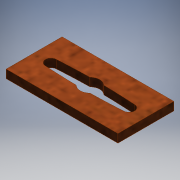
# Autodesk Inventor part: acople madera
Saved by Autodesk Inventor 2016 (Build 200138000, 138)
## iProperties
Created: 2016-08-02
Part Number: acople madera
Material: Madera (nogal)
Document SubType Name: Modeling
Designer: DanielFelipe
Density: 0.55 g/cm^3
Appearance: Nogal - Natural pulido
Mass: 1.07378 g
Surface Area: 18.7068 cm^2
Volume: 1.95232 cm^3
Author: DanielFelipe
Autodesk Inventor part; units mm, degrees
ref_plane "YZ Plane" through (0, 0, 0) normal (1, 0, 0) x (0, 1, 0)
ref_plane "XZ Plane" through (0, 0, 0) normal (0, 1, 0) x (-1, 0, 0)
ref_plane "XY Plane" through (0, 0, 0) normal (0, 0, 1) x (1, 0, 0)
sketch "Boceto1" plane through (0, 0, 0) normal (0, 0, 1) x (1, 0, 0)
  arc A0 (-2.4791, 2.4706) -> (-14, 2) centre (1.6231, -239.1959) ccw
  arc A1 (-14, 2) -> (-14, -2) centre (-14, 0) ccw
  arc A2 (-14, -2) -> (-2.4791, -2.4706) centre (1.6231, 239.1959) ccw
  arc A3 (2.4791, -2.4706) -> (14, -2) centre (-1.6231, 239.1959) ccw
  arc A4 (14, -2) -> (14, 2) centre (14, 0) ccw
  arc A5 (14, 2) -> (2.4791, 2.4706) centre (-1.6231, -239.1959) ccw
  line L0 (-20, -10) -> (20, -10)
  line L1 (20, -10) -> (20, 10)
  line L2 (20, 10) -> (-20, 10)
  line L3 (-20, 10) -> (-20, -10)
  line L4 (-20, -10) -> (20, 10) construction
  line L5 (20, -10) -> (-20, 10) construction
  arc A6 (-2.4791, -2.4706) -> (2.4791, -2.4706) centre (0, 0) ccw
  arc A7 (2.4791, 2.4706) -> (-2.4791, 2.4706) centre (0, 0) ccw
  line L6 (-4.8381, 2.4191) -> (-4.8381, -2.4191)
  line L7 (4.8381, -2.4191) -> (2.4791, 2.4706)
  dimension "d2" = 40
  constraints: 20 point on circle, 16 end point, 8 centre point, 2 midpoint, 2 parallel, 2 point on line, 1 horizontal, 1 perpendicular
  measures "d2" distance of L2.end L1.end
extrude "Extrusión1" add sketch "Boceto1" along normal blind 3
